Under Camera (Autodesk Fusion 360 design; units mm, degrees)
Autodesk Fusion 360 part; units mm, degrees
note: some values were not read from the file. Chosen so that the rebuilt part matches the saved one: which face or edge a step refers to. Set by a fixed rule: which sketch regions a step uses.
sketch "Sketch1" plane through (0, -227.1998, 566.5) normal (1, 0, 0) x (0, 1, 0) in component "Under Cam"
  line L0 (-26, -3.5) -> (12.5005, -3.5)
  line L1 (12.5005, -3.5) -> (8.0001, -24)
  line L2 (8.0001, -24) -> (-15.3, -24)
  line L3 (-15.3, -24) -> (-15.3, -28.1777)
  line L4 (-15.3, -28.1777) -> (-17, -28.1777)
  line L5 (-17, -28.1777) -> (-26, -3.5)
  line L6 (3.7005, -3.5) -> (3.7005, -24) construction
  circle A0 centre (3.7005, -8.5) radius 0.75
  circle A1 centre (3.7005, -18.5) radius 0.75
  dimension "d282" = 8.8
  dimension "d283" = 1.5
  dimension "d284" = 5
  dimension "d285" = 1.5
  dimension "d286" = 10
  constraint horizontal L0
  constraint parallel L0 L2
  constraint perpendicular L2 L3
  constraint perpendicular L3 L4
  constraint coincident L0 L6.start
  constraint coincident L2 L6.end
  constraint perpendicular L2 L6
  constraint coincident L6 A0.centre
  constraint coincident L6 A1.centre
  measures "d282" distance of L0.end L6.start
  measures "d283" diameter of A0
  measures "d284" distance of L0 A0.centre
  measures "d285" diameter of A1
  measures "d286" distance of A0.centre A1.centre
extrude "Extrude1" add sketch "Sketch1" against normal blind 24 contours L0 L1 L2 L3 L4 L5 | A0 | A1 makes body 1 in component "Under Cam"
ref_plane "WorkPlane2" through (-12, -257.4998, 540.4111) normal (0, 1, 0) x (0, 0, -1) in component "Under Cam"
sketch "Sketch2" plane through (-71.456, -257.4998, 540.4111) normal (0, 1, 0) x (1, 0, 0) in component "Under Cam"
  line L0 (71.456, 2.0889) -> (71.456, -22.5888)
  line L1 (71.456, -22.5888) -> (47.456, -22.5888)
  line L2 (47.456, -22.5888) -> (47.456, 2.0889)
  line L3 (47.456, 2.0889) -> (71.456, 2.0889)
  line L4 (49.456, -21.5888) -> (69.456, -21.5888)
  line L5 (69.456, -21.5888) -> (69.456, 2.0889)
  line L6 (69.456, 2.0889) -> (49.456, 2.0889)
  line L7 (49.456, 2.0889) -> (49.456, -21.5888)
  dimension "d273" = 2
  dimension "d274" = 2
  dimension "d275" = 1
  constraint horizontal L4
  constraint vertical L5
  constraint horizontal L6
  constraint vertical L7
  constraint coincident L3 L5.end
  measures "d273" horizontal distance of L1.end L4.start
  measures "d274" horizontal distance of L0.end L4.end
  measures "d275" vertical distance of L0.end L4.end
extrude "Extrude2" cut sketch "Sketch2" along normal blind 13 contours L3 L4 L5 L6 L7 bodies 1 in component "Under Cam"
extrude "Extrude4" cut sketch "Sketch1" against normal blind 10 contours A0 | A1 bodies 1 in component "Under Cam"
sketch "Sketch3" plane through (0, -227.1998, 566.5) normal (1, 0, 0) x (0, 1, 0) in component "Under Cam"
  line L0 (-1.8995, -3.5) -> (9.3005, -3.5)
  line L1 (9.3005, -3.5) -> (9.3005, -49)
  line L2 (9.3005, -49) -> (-1.8995, -49)
  line L3 (-1.8995, -49) -> (-1.8995, -3.5)
  line L4 (-26, -3.5) -> (12.5005, -3.5)
  line L5 (-26, -3.5) -> (12.5005, -3.5) construction
  line L6 (3.7005, -3.5) -> (3.7005, -49) construction
  circle A0 centre (3.7005, -8.5) radius 1.1
  circle A1 centre (3.7005, -18.5) radius 1.1
  line L7 (3.7005, -49) -> (3.7005, -77.9127) construction
  point P0 (3.7005, -8.5)
  point P1 (3.7005, -18.5)
  dimension "d278" = 11.2
  dimension "d281" = 8.8
  dimension "d289" = 2.2
  dimension "d290" = 2.2
  constraint horizontal L0
  constraint vertical L1
  constraint horizontal L2
  constraint vertical L3
  constraint coincident L4.start L5.start
  constraint coincident L4.end L5.end
  constraint coincident L0.end L5
  constraint midpoint L0 L6.start
  constraint perpendicular L0 L6
  constraint coincident P0 A0.centre
  constraint coincident P1 A1.centre
  constraint perpendicular L2 L7
  measures "d278" distance of L0.start L0.end
  measures "d281" distance of L4.end L6.start
  measures "d289" diameter of A0
  measures "d290" diameter of A1
extrude "Extrude3" add sketch "Sketch3" along normal blind 5 separate body makes body 2 in component "Under Cam"
sketch "Sketch4" plane through (5, 0, 0) normal (1, 0, 0) x (0, 1, 0) in component "Under Cam"
  circle A0 centre (-223.4993, 548) radius 1.1
  circle A1 centre (-223.4993, 558) radius 1.1
  line L0 (-229.0993, 517.5) -> (-217.8993, 517.5)
  line L1 (-217.8993, 517.5) -> (-217.8993, 563)
  line L2 (-217.8993, 563) -> (-229.0993, 563)
  line L3 (-229.0993, 563) -> (-229.0993, 517.5)
  circle A2 centre (-223.4993, 558) radius 2.5
  circle A3 centre (-223.4993, 548) radius 2.5
  line L4 (-223.4993, 548) -> (-223.4993, 517.5) construction
  dimension "d291" = 5
  dimension "d292" = 5
  constraint concentric A1 A2
  constraint concentric A0 A3
  constraint coincident A0.centre A3.centre
  constraint midpoint L0 L4.end
  measures "d291" diameter of A2
  measures "d292" diameter of A3
sketch "Sketch6" plane through (0, -227.1998, 566.5) normal (1, 0, 0) x (0, 1, 0) in component "Under Cam"
  line L0 (-1.8995, -49) -> (9.3005, -49)
  line L1 (3.7005, -49) -> (3.7005, -32.5726) construction
  circle A0 centre (3.7005, -54.5726) radius 22
  circle A1 centre (3.7005, -54.5726) radius 21
  circle A2 centre (3.7005, -54.5726) radius 13.5
  circle A3 centre (3.7005, -54.5726) radius 12.5
  line L2 (9.3005, -49) -> (9.3005, -33.2972)
  line L3 (-1.8995, -49) -> (-1.8995, -33.2972)
  circle A4 centre (3.7005, -37) radius 0.75
  circle A5 centre (3.7005, -44) radius 0.75
  point P0 (9.3005, -49)
  point P1 (-1.8995, -49)
  dimension "d295" = 44
  dimension "d298" = -1
  dimension "d299" = -8.5
  dimension "d300" = -9.5
  dimension "d305" = 1.5
  dimension "d306" = 1.5
  dimension "d307" = 5
  dimension "d308" = 7
  constraint coincident P1 L0.start
  constraint coincident P0 L0.end
  constraint midpoint L0 L1.start
  constraint perpendicular L0 L1
  constraint coincident L1 A0.centre
  constraint coincident A0 L2.end
  constraint vertical L2
  constraint coincident A0 L3.end
  constraint perpendicular L0 L3
  constraint coincident L1.end A0
  constraint coincident L1 A4.centre
  constraint coincident L1 A5.centre
  measures "d295" diameter of A0
  measures "d305" diameter of A4
  measures "d306" diameter of A5
  measures "d307" distance of L1.start A5.centre
  measures "d308" distance of A4.centre A5.centre
extrude "Extrude6" add sketch "Sketch6" against normal blind 36.5 separate body contours L0 A3 L2 L3 | L0 A3 L2 L3 | A2 A3 L2 L3 | A2 A3 L2 L3 | A1 A2 L2 L3 | A1 A2 L2 L3 | A0 A1 L2 L3 | A0 A1 L2 L3 | A4 | A5 makes body 3 in component "Under Cam"
extrude "Extrude7" cut sketch "Sketch6" against normal blind 10 contours L0 A3 L2 L3 | A1 A2 L2 L3 picked at (3.532, -55.0208) picked at (-4.7622, -38.1727) bodies 3 in component "Under Cam"
extrude "Extrude8" add sketch "Sketch6" along normal blind 2.5 contours A2 A3 L2 L3 | A0 A1 L2 L3 picked at (-3.0056, -43.6595) picked at (-3.9032, -34.6912) bodies 3 in component "Under Cam"
extrude "Extrude9" cut sketch "Sketch6" against normal blind 10 contours A4 | A5 bodies 3 in component "Under Cam"
sketch "Sketch7" plane through (5, 0, 0) normal (1, 0, 0) x (0, 1, 0) in component "Under Cam"
  line L0 (-229.0993, 517.5) -> (-217.8993, 517.5)
  line L1 (-217.8993, 517.5) -> (-217.8993, 563)
  line L2 (-217.8993, 563) -> (-229.0993, 563)
  line L3 (-229.0993, 563) -> (-229.0993, 517.5)
  circle A0 centre (-223.4993, 529.5) radius 1.1
  circle A1 centre (-223.4993, 522.5) radius 1.1
  circle A2 centre (-223.4993, 529.5) radius 2.5
  circle A3 centre (-223.4993, 522.5) radius 2.5
  circle A4 centre (-223.4993, 558) radius 1.1
  circle A5 centre (-223.4993, 548) radius 1.1
  point P0 (-223.4993, 529.5)
  point P1 (-223.4993, 522.5)
  dimension "d311" = 2.2
  dimension "d312" = 2.2
  dimension "d313" = 5
  dimension "d314" = 5
  constraint coincident P0 A0.centre
  constraint coincident P1 A1.centre
  constraint concentric A0 A2
  constraint concentric A1 A3
  measures "d311" diameter of A0
  measures "d312" diameter of A1
  measures "d313" diameter of A2
  measures "d314" diameter of A3
extrude "Extrude5" cut sketch "Sketch4" sketch "Sketch7" against normal blind 2.5 contours A2 | A3 of sketch 2 contours A2 | A3 bodies 2 in component "Under Cam"
extrude "Extrude10" cut sketch "Sketch7" against normal blind 5 contours A0 | A1 bodies 2 in component "Under Cam"
sketch "Sketch8" plane through (0, 0, 563) normal (0, 0, 1) x (-1, 0, 0) in component "Under Cam"
  line L0 (0, 253.1998) -> (0, 214.6993)
  line L1 (0, 214.6993) -> (24, 214.6993)
  line L2 (24, 214.6993) -> (24, 253.1998)
  line L3 (24, 253.1998) -> (0, 253.1998)
  line L4 (12, 214.6993) -> (12, 253.1998) construction
  circle A0 centre (12, 226.9495) radius 0.75
  circle A1 centre (12, 240.9495) radius 0.75
  line L5 (12, 233.9495) -> (0, 233.9495) construction
  dimension "d389" = 1.5
  dimension "d390" = 1.5
  dimension "d391" = 7
  dimension "d392" = 7
  constraint midpoint L1 L4.start
  constraint midpoint L3 L4.end
  constraint coincident L4 A0.centre
  constraint coincident L4 A1.centre
  constraint midpoint L4 L5.start
  constraint midpoint L0 L5.end
  measures "d389" diameter of A0
  measures "d390" diameter of A1
  measures "d391" distance of A1.centre L5.start
  measures "d392" distance of A0.centre L5.start
extrude "Extrude11" cut sketch "Sketch8" against normal blind 10 contours A0 | A1 bodies 1 in component "Under Cam"
component "Under Cam" placed x (1, 0, 0) y (0, 1, 0) z (0, 0, 1) at (0, 0, 0)
equation "Trous_Vis_diam2 = 2.2 mm"
named bodies: "support double cam", "fixation latérale", "Cylindre"
